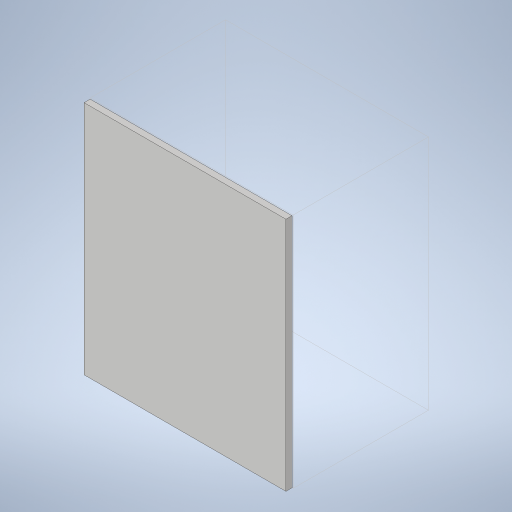
# Autodesk Inventor part: Simple door Skeleton
Saved by Autodesk Inventor 2024 (Build 280153000, 153)
## iProperties
Created: 2017-04-10
Part Number: Simple door Skeleton
Material: Generic
Document SubType Name: Modeling
Designer: SvetlanaB
Density: 1 g/cm^3
Appearance: Default
Description: Simple door Skeleton
Panel_thickness: 18,000 mm
Type: 1,000 ul
Front_offset: 2,000 mm
Width: 600,000 mm
Depth: 400,000 mm
Height: 700,000 mm
Top_offset: 1,500 mm
Bottom_offset: 1,500 mm
Left_offset: 1,500 mm
Right_offset: 1,500 mm
Author: SvetlanaB
Autodesk Inventor part; units mm, degrees
ref_plane "YZ Plane" through (0, 0, 0) normal (1, 0, 0) x (0, 1, 0)
ref_plane "XZ Plane" through (0, 0, 0) normal (0, 1, 0) x (-1, 0, 0)
ref_plane "XY Plane" through (0, 0, 0) normal (0, 0, 1) x (1, 0, 0)
sketch "Sketch1" plane through (0, 0, 0) normal (0, 0, 1) x (1, 0, 0)
  line L0 (-300, 200) -> (300, 200)
  line L1 (300, 200) -> (300, -200)
  line L2 (300, -200) -> (-300, -200)
  line L3 (-300, -200) -> (-300, 200)
  line L4 (-300, 200) -> (300, -200) construction
  line L5 (300, 200) -> (-300, -200) construction
  point P0 (0, 0)
  dimension "Width" = 600
  dimension "Depth" = 400
  constraints: 12 end point, 2 midpoint, 2 parallel, 1 horizontal, 1 perpendicular
  measures "Width" distance of L1.end L2.end
  measures "Depth" distance of L0.end L1.end
extrude "Extrusion1" add sketch "Sketch1" along normal mid plane 700
sketch "Sketch2" plane through (-300, -200, 350) normal (0, -1, 0) x (1, 0, 0)
  line L0 (600, 0) -> (600, -700) projected
  line L1 (0, 0) -> (600, 0) projected
  line L2 (0, 0) -> (0, -700) projected
  line L3 (600, -700) -> (0, -700) projected
  point P0 (300, -350)
extrude "Extrusion2" add sketch "Sketch2" against normal blind 18 separate body
sketch "Sketch4" plane through (-300, -200, 350) normal (0, -1, 0) x (1, 0, 0)
  line L0 (600, -700) -> (600, 0) construction
  line L1 (600, 0) -> (0, 0) construction
  line L2 (0, 0) -> (0, -700) construction
  line L3 (0, -700) -> (600, -700) construction
  line L4 (1.5, -1.5) -> (598.5, -1.5)
  line L5 (598.5, -1.5) -> (598.5, -698.5)
  line L6 (598.5, -698.5) -> (1.5, -698.5)
  line L7 (1.5, -698.5) -> (1.5, -1.5)
  point P0 (300, -350)
  dimension "Top_offset" = 1.5
  dimension "Bottom_offset" = 1.5
  dimension "Left_offset" = 1.5
  dimension "Right_offset" = 1.5
  constraints: 8 end point, 2 parallel, 1 horizontal, 1 perpendicular
  measures "Top_offset" distance between parallel lines of L4 L1
  measures "Bottom_offset" distance between parallel lines of L3 L6
  measures "Left_offset" distance between parallel lines of L7 L2
  measures "Right_offset" distance between parallel lines of L0 L5
extrude "Extrusion3" cut sketch "Sketch4" against normal through all keep common part bodies 2
move or copy body "Move1" bodies to move or copy 2 copy no translate (0, -20, 0)
equation "\"d4\" = Panel_thickness"
equation "\"d8\" = -Panel_thickness - Front_offset"
equation "\"Panel_thickness\" = 18"
equation "\"Front_offset\" = 2"
